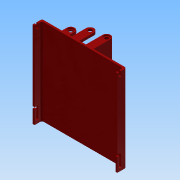
# Autodesk Inventor part: 电机座
Saved by Autodesk Inventor 2015 (Build 190159000, 159)
## iProperties
Created: 2017-05-27
Part Number: 电机座
Material: 常规
Document SubType Name: Modeling
Designer: Administrator
Density: 1 g/cm^3
Appearance: 红
Author: Administrator
Autodesk Inventor part; units mm, degrees
ref_plane "YZ Plane" through (0, 0, 0) normal (1, 0, 0) x (0, 1, 0)
ref_plane "XZ Plane" through (0, 0, 0) normal (0, 1, 0) x (-1, 0, 0)
ref_plane "XY Plane" through (0, 0, 0) normal (0, 0, 1) x (1, 0, 0)
sketch "草图1" plane through (0, 0, 0) normal (0, 0, 1) x (1, 0, 0)
  line L0 (-230, 0) -> (230, 0)
  line L1 (230, 0) -> (230, 50)
  line L2 (230, 50) -> (-230, 50)
  line L3 (-230, 50) -> (-230, 0)
  line L4 (-220, 0) -> (220, 0)
  line L5 (220, 0) -> (220, 40)
  line L6 (220, 40) -> (-220, 40)
  line L7 (-220, 40) -> (-220, 0)
  point P0 (0, 0)
  point P1 (0, 0)
  dimension "d0" = 10
  dimension "d1" = 10
  dimension "d2" = 10
  dimension "d3" = 460
  dimension "d4" = 40
  constraints: 16 end point, 4 parallel, 2 horizontal, 2 perpendicular, 1 coincident, 1 midpoint, 1 point on line
  measures "d0" distance between parallel lines of L6 L2
  measures "d1" distance between parallel lines of L1 L5
  measures "d2" distance between parallel lines of L3 L7
  measures "d3" distance of L1.end L2.end
  measures "d4" distance between parallel lines of L0 L6
extrude "拉伸1" add sketch "草图1" along normal blind 469.5 contours L3 L2 L1 L0 L5 L6 L7
fillet "圆角1" radius 10 4 edges at (230, 50, 234.75) (-230, 50, 234.75) (-220, 40, 234.75) (220, 40, 234.75)
sketch "草图2" plane through (-220, 50, 0) normal (0, 1, 0) x (1, 0, 0)
  line L0 (34, -391.5) -> (76, -391.5)
  line L1 (76, -391.5) -> (76, -405.5)
  line L2 (76, -405.5) -> (34, -405.5)
  line L3 (34, -405.5) -> (34, -391.5)
  line L4 (-10, 0) -> (-10, -469.5) projected
  line L5 (440, -469.5) -> (0, -469.5) projected
  point P0 (220, 0)
  dimension "d8" = 42
  dimension "d9" = 14
  dimension "d10" = 44
  dimension "d11" = 64
  constraints: 8 end point, 2 parallel, 1 horizontal, 1 perpendicular
  measures "d8" distance of L1.end L2.end
  measures "d9" distance of L2.end L0.start
  measures "d10" distance between parallel lines of L4 L3
  measures "d11" distance between parallel lines of L5 L2
extrude "拉伸2" add sketch "草图2" along normal blind 112.384
fillet "圆角2" radius 21 2 edges at (-144, 162.384, 398.5) (-186, 162.384, 398.5)
sketch "草图3" plane through (-186, 50, 405.5) normal (0, 0, 1) x (1, 0, 0)
  circle A0 centre (21, 91.384) radius 16
  arc A1 (42, 91.384) -> (0, 91.384) centre (21, 91.384) ccw projected
  point P0 (186, -50)
  dimension "d15" = 32
  constraints: 1 centre point, 1 concentric
  measures "d15" diameter of A0
extrude "拉伸3" cut sketch "草图3" against normal blind 7
sketch "草图4" plane through (-165, 141.384, 398.5) normal (0, 0, 1) x (1, 0, 0)
  circle A0 centre (0, 0) radius 12
  point P0 (165, -141.384)
  dimension "d18" = 24
  constraints: 1 centre point
  measures "d18" diameter of A0
extrude "拉伸4" cut sketch "草图4" against normal blind 3
sketch "草图5" plane through (-165, 141.384, 395.5) normal (0, 0, 1) x (1, 0, 0)
  circle A0 centre (0, 0) radius 10.5
  point P0 (165, -141.384)
  dimension "d21" = 21
  constraints: 1 centre point
  measures "d21" diameter of A0
extrude "拉伸5" cut sketch "草图5" against normal blind 4
sketch "草图6" plane through (-220, 50, 0) normal (0, 1, 0) x (1, 0, 0)
  line L0 (139, -442) -> (181, -442)
  line L1 (181, -442) -> (181, -456)
  line L2 (181, -456) -> (139, -456)
  line L3 (139, -456) -> (139, -442)
  line L4 (440, -469.5) -> (0, -469.5) projected
  line L5 (-10, 0) -> (-10, -469.5) projected
  point P0 (220, 0)
  dimension "d24" = 42
  dimension "d25" = 14
  dimension "d26" = 13.5
  dimension "d27" = 149
  constraints: 8 end point, 2 parallel, 1 horizontal, 1 perpendicular
  measures "d24" distance of L1.end L2.end
  measures "d25" distance of L0.end L1.end
  measures "d26" distance between parallel lines of L4 L2
  measures "d27" distance between parallel lines of L5 L3
extrude "拉伸6" add sketch "草图6" along normal blind 112.384
fillet "圆角3" radius 21 2 edges at (-39, 162.384, 449) (-81, 162.384, 449)
sketch "草图7" plane through (-39, 50, 442) normal (0, 0, -1) x (-1, 0, 0)
  circle A0 centre (21, 91.384) radius 16
  arc A1 (42, 91.384) -> (0, 91.384) centre (21, 91.384) ccw projected
  point P0 (-39, -50)
  dimension "d31" = 32
  constraints: 1 centre point, 1 concentric
  measures "d31" diameter of A0
extrude "拉伸7" cut sketch "草图7" against normal blind 7
sketch "草图8" plane through (-60, 141.384, 449) normal (0, 0, -1) x (-1, 0, 0)
  circle A0 centre (0, 0) radius 13
  circle A1 centre (0, 0) radius 16 projected
  point P0 (-60, -141.384)
  dimension "d34" = 26
  constraints: 1 centre point, 1 concentric
  measures "d34" diameter of A0
extrude "拉伸8" cut sketch "草图8" against normal blind 3 contours A0
sketch "草图9" plane through (-60, 141.384, 452) normal (0, 0, -1) x (-1, 0, 0)
  circle A0 centre (0, 0) radius 10.5
  circle A1 centre (0, 0) radius 13 projected
  point P0 (-60, -141.384)
  dimension "d37" = 21
  constraints: 1 centre point, 1 concentric
  measures "d37" diameter of A0
extrude "拉伸9" cut sketch "草图9" against normal blind 4 contours A0
sketch "草图10" plane through (-220, 50, 0) normal (0, 1, 0) x (1, 0, 0)
  line L0 (120, -209) -> (200, -209)
  line L1 (200, -209) -> (200, -223)
  line L2 (200, -223) -> (120, -223)
  line L3 (120, -223) -> (120, -209)
  line L4 (-10, 0) -> (-10, -469.5) projected
  line L5 (440, -469.5) -> (0, -469.5) projected
  point P0 (220, 0)
  dimension "d40" = 80
  dimension "d41" = 14
  dimension "d42" = 130
  dimension "d43" = 246.5
  constraints: 8 end point, 2 parallel, 1 horizontal, 1 perpendicular
  measures "d40" distance of L1.end L2.end
  measures "d41" distance of L2.end L0.start
  measures "d42" distance between parallel lines of L4 L3
  measures "d43" distance between parallel lines of L5 L2
extrude "拉伸10" add sketch "草图10" along normal blind 91.384
sketch "草图12" plane through (-100, 50, 223) normal (0, 0, 1) x (1, 0, 0)
  line L0 (80, 91.384) -> (0, 91.384) projected
  circle A0 centre (40, 91.384) radius 21
  point P0 (100, -50)
  dimension "d47" = 42
  constraints: 1 centre point, 1 midpoint
  measures "d47" diameter of A0
extrude "拉伸11" cut sketch "草图12" against normal blind 7
sketch "草图13" plane through (-100, 50, 216) normal (0, 0, 1) x (1, 0, 0)
  line L0 (80, 91.384) -> (0, 91.384) projected
  circle A0 centre (40, 91.384) radius 17
  circle A1 centre (40, 91.384) radius 16 projected
  point P0 (100, -50)
  dimension "d50" = 34
  constraints: 1 centre point, 1 concentric, 1 midpoint
  measures "d50" diameter of A0
extrude "拉伸12" cut sketch "草图13" against normal blind 2
sketch "草图14" plane through (-100, 50, 214) normal (0, 0, 1) x (1, 0, 0)
  circle A0 centre (40, 91.384) radius 15.5
  circle A1 centre (40, 91.384) radius 10.5 projected
  point P0 (100, -50)
  dimension "d53" = 31
  constraints: 1 centre point, 1 concentric
  measures "d53" diameter of A0
extrude "拉伸13" cut sketch "草图14" against normal through all contours A0 | A1
sketch "草图15" plane through (-220, 141.384, 0) normal (0, 1, 0) x (1, 0, 0)
  circle A0 centre (193, -216) radius 2.5
  circle A1 centre (127, -216) radius 2.5
  line L0 (200, -223) -> (200, -209) projected
  line L1 (200, -209) -> (175.5, -209) projected
  line L2 (144.5, -209) -> (120, -209) projected
  line L3 (120, -209) -> (120, -223) projected
  point P0 (220, 0)
  dimension "d56" = 5
  dimension "d57" = 5
  dimension "d58" = 7
  dimension "d59" = 7
  dimension "d60" = 7
  dimension "d61" = 7
  constraints: 2 centre point
  measures "d56" diameter of A0
  measures "d57" diameter of A1
  measures "d58" distance from line of L0 A0.centre
  measures "d59" distance from line of L1 A0.centre
  measures "d60" distance from line of L2 A1.centre
  measures "d61" distance from line of L3 A1.centre
extrude "拉伸14" cut sketch "草图15" against normal blind 15
thread "螺纹1" size "M5x0.8" class "6H" standard "ANSI Metric M Profile" full length
thread "螺纹2" size "M5x0.8" class "6H" standard "ANSI Metric M Profile" full length
sketch "草图16" plane through (-220, 50, 0) normal (0, 1, 0) x (1, 0, 0)
  line L0 (229, -349.5) -> (271, -349.5)
  line L1 (271, -349.5) -> (271, -469.5)
  line L2 (271, -469.5) -> (229, -469.5)
  line L3 (229, -469.5) -> (229, -349.5)
  line L4 (440, -469.5) -> (0, -469.5) projected
  line L5 (-10, 0) -> (-10, -469.5) projected
  point P0 (220, 0)
  dimension "d68" = 42
  dimension "d69" = 120
  dimension "d70" = 0
  dimension "d71" = 239
  constraints: 8 end point, 2 parallel, 1 horizontal, 1 perpendicular
  measures "d68" distance of L0.start L0.end
  measures "d69" distance of L2.end L0.start
  measures "d70" distance between parallel lines of L4 L2
  measures "d71" distance between parallel lines of L5 L3
extrude "拉伸15" add sketch "草图16" along normal blind 112.384
fillet "圆角5" radius 21 2 edges at (51, 162.384, 409.5) (9, 162.384, 409.5)
sketch "草图17" plane through (9, 50, 469.5) normal (0, 0, 1) x (-1, 0, 0)
  circle A0 centre (-21, -91.384) radius 16
  arc A1 (-42, -91.384) -> (0, -91.384) centre (-21, -91.384) ccw projected
  point P0 (9, 50)
  dimension "d75" = 32
  constraints: 1 centre point, 1 concentric
  measures "d75" diameter of A0
extrude "拉伸16" cut sketch "草图17" against normal blind 7
sketch "草图18" plane through (51, 50, 349.5) normal (0, 0, -1) x (-1, 0, 0)
  circle A0 centre (21, 91.384) radius 16
  arc A1 (42, 91.384) -> (0, 91.384) centre (21, 91.384) ccw projected
  point P0 (51, -50)
  dimension "d78" = 32
  constraints: 1 centre point, 1 concentric
  measures "d78" diameter of A0
extrude "拉伸17" cut sketch "草图18" against normal blind 7
sketch "草图19" plane through (30, 141.384, 356.5) normal (0, 0, -1) x (-1, 0, 0)
  circle A0 centre (0, 0) radius 10.5
  arc A1 (21, 0) -> (-21, 0) centre (0, 0) ccw projected
  point P0 (30, -141.384)
  dimension "d81" = 21
  constraints: 1 centre point, 1 concentric
  measures "d81" diameter of A0
extrude "拉伸18" cut sketch "草图19" against normal through all
sketch "草图20" plane through (-220, 50, 0) normal (0, 1, 0) x (1, 0, 0)
  line L0 (259, -262) -> (301, -262)
  line L1 (301, -262) -> (301, -276)
  line L2 (301, -276) -> (259, -276)
  line L3 (259, -276) -> (259, -262)
  line L4 (440, -469.5) -> (0, -469.5) projected
  line L5 (-10, 0) -> (-10, -469.5) projected
  point P0 (220, 0)
  dimension "d84" = 42
  dimension "d85" = 14
  dimension "d86" = 193.5
  dimension "d87" = 269
  constraints: 8 end point, 2 parallel, 1 horizontal, 1 perpendicular
  measures "d84" distance of L1.end L2.end
  measures "d85" distance of L0.end L1.end
  measures "d86" distance between parallel lines of L4 L2
  measures "d87" distance between parallel lines of L5 L3
extrude "拉伸19" add sketch "草图20" along normal blind 112.384
fillet "圆角6" radius 21 2 edges at (81, 162.384, 269) (39, 162.384, 269)
sketch "草图23" plane through (81, 50, 262) normal (0, 0, -1) x (-1, 0, 0)
  circle A0 centre (21, 91.384) radius 16
  arc A1 (42, 91.384) -> (0, 91.384) centre (21, 91.384) ccw projected
  point P0 (81, -50)
  dimension "d91" = 32
  constraints: 1 centre point, 1 concentric
  measures "d91" diameter of A0
extrude "拉伸20" cut sketch "草图23" against normal blind 7
sketch "草图24" plane through (60, 141.384, 269) normal (0, 0, -1) x (-1, 0, 0)
  circle A0 centre (0, 0) radius 14
  circle A1 centre (0, 0) radius 16 projected
  point P0 (60, -141.384)
  dimension "d94" = 28
  constraints: 1 centre point, 1 concentric
  measures "d94" diameter of A0
extrude "拉伸21" cut sketch "草图24" against normal blind 3 contours A0
sketch "草图25" plane through (60, 141.384, 272) normal (0, 0, -1) x (-1, 0, 0)
  circle A0 centre (0, 0) radius 10.5
  circle A1 centre (0, 0) radius 14 projected
  point P0 (60, -141.384)
  dimension "d97" = 21
  constraints: 1 centre point, 1 concentric
  measures "d97" diameter of A0
extrude "拉伸22" cut sketch "草图25" against normal blind 4 contours A0
sketch "草图26" plane through (-220, 50, 0) normal (0, 1, 0) x (1, 0, 0)
  circle A0 centre (205, -30) radius 5
  circle A1 centre (355, -30) radius 5
  circle A2 centre (205, -150) radius 5
  circle A3 centre (355, -150) radius 5
  line L0 (430, 0) -> (10, 0) projected
  line L1 (450, -469.5) -> (450, 0) projected
  point P0 (220, 0)
  dimension "d100" = 10
  dimension "d101" = 10
  dimension "d102" = 10
  dimension "d103" = 10
  dimension "d104" = 30
  dimension "d105" = 30
  dimension "d106" = 150
  dimension "d107" = 150
  dimension "d108" = 95
  dimension "d109" = 245
  dimension "d110" = 95
  dimension "d111" = 245
  constraints: 4 centre point
  measures "d100" diameter of A0
  measures "d101" diameter of A1
  measures "d102" diameter of A2
  measures "d103" diameter of A3
  measures "d104" distance from line of L0 A0.centre
  measures "d105" distance from line of L0 A1.centre
  measures "d106" distance from line of L0 A3.centre
  measures "d107" distance from line of L0 A2.centre
  measures "d108" distance from line of L1 A3.centre
  measures "d109" distance from line of L1 A2.centre
  measures "d110" distance from line of L1 A1.centre
  measures "d111" distance from line of L1 A0.centre
extrude "拉伸23" add sketch "草图26" along normal blind 20
thread "螺纹3" size "M10x1.5" class "6g" standard "ANSI Metric M Profile" full length
thread "螺纹4" size "M10x1.5" class "6g" standard "ANSI Metric M Profile" full length
thread "螺纹5" size "M10x1.5" class "6g" standard "ANSI Metric M Profile" full length
thread "螺纹6" size "M10x1.5" class "6g" standard "ANSI Metric M Profile" full length
chamfer "倒角1" distance 1 angle 45 4 edges at (-20, 70, 30) (130, 70, 30) (130, 70, 150) (-20, 70, 150)
sketch "草图28" plane through (230, 0, 469.5) normal (1, 0, 0) x (0, 0, -1)
  circle A0 centre (20, 15) radius 5
  line L0 (469.5, 0) -> (0, 0) projected
  line L1 (0, 0) -> (0, 40) projected
  line L2 (20, 10) -> (0, 10)
  line L3 (0, 10) -> (0, 20)
  line L4 (0, 20) -> (20, 20)
  line L5 (20, 20) -> (20, 10)
  circle A1 centre (449.5, 15) radius 5
  line L6 (469.5, 0) -> (469.5, 40) projected
  line L7 (449.5, 10) -> (385.5, 10)
  line L8 (385.5, 10) -> (385.5, 20)
  line L9 (385.5, 20) -> (449.5, 20)
  line L10 (449.5, 20) -> (449.5, 10)
  arc A2 (390.5, 20) -> (385.5, 15) centre (390.5, 15) ccw
  line L11 (469.5, 0) -> (0, 0) projected
  line L12 (385.5, 10) -> (395.5, 10)
  line L13 (395.5, 10) -> (395.5, 0)
  line L14 (395.5, 0) -> (385.5, 0)
  line L15 (385.5, 0) -> (385.5, 10)
  dimension "d140" = 10
  dimension "d143" = 10
  dimension "d141" = 15
  dimension "d142" = 20
  dimension "d144" = 15
  dimension "d145" = 20
  dimension "d146" = 64
  dimension "d147" = 10
  constraints: 24 end point, 6 horizontal, 6 parallel, 3 perpendicular, 2 midpoint, 2 point on circle, 2 point on line, 2 tangent, 2 vertical alignment, 1 centre point, 4 other
  measures "d141" distance from line of L0 point (20, 15)
  measures "d142" distance from line of L1 point (20, 15)
  measures "d144" distance from line of L0 point (449.5, 15)
  measures "d145" distance from line of L6 point (449.5, 15)
  measures "d146" distance of L8.end L9.end
  measures "d147" distance of L13.end L14.end
extrude "拉伸26" cut sketch "草图28" against normal through all contours A0 L5 | L5 A0 | A0 L2 L1 L4 | L0 L15 L7 L13 | L7 L8 A2 L9 A1 | L10 A1 | A1 L10
equation "\"d54\" = d53"
